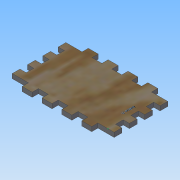
# Autodesk Inventor part: WallToWall(Perpendicular1)
Saved by Autodesk Inventor 2015 (Build 190159000, 159)
## iProperties
Created: 2014-11-11
Part Number: WallToWall(Perpendicular1)
Material: Generic
Document SubType Name: Modeling
Designer: 0
Density: 1 g/cm^3
Appearance: Default
Mass: 72.7404 g
Surface Area: 272.974 cm^2
Volume: 72.7404 cm^3
Author: 0
Autodesk Inventor part; units mm, degrees
ref_plane "YZ Plane" through (0, 0, 0) normal (1, 0, 0) x (0, 1, 0)
ref_plane "XZ Plane" through (0, 0, 0) normal (0, 1, 0) x (-1, 0, 0)
ref_plane "XY Plane" through (0, 0, 0) normal (0, 0, 1) x (1, 0, 0)
sketch "Sketch1" plane through (0, 0, 0) normal (0, 1, 0) x (-1, 0, 0)
  line L0 (0, 0) -> (127, 0)
  line L1 (127, 0) -> (127, -76.2)
  line L2 (127, -76.2) -> (0, -76.2)
  line L3 (0, -76.2) -> (0, 0)
  dimension "BoxHeight" = 127
  dimension "d1" = 76.2
  constraints: 8 end point, 2 parallel, 1 coincident, 1 horizontal, 1 perpendicular
  measures "BoxHeight" distance of L1.end L2.end
  measures "d1" distance of L0.end L1.end
sketch "Sketch2" plane through (0, 0, 0) normal (0, 1, 0) x (-1, 0, 0)
  line L0 (0, 0) -> (-8.89, 0)
  line L1 (-8.89, 0) -> (-8.89, -10.8857)
  line L2 (-8.89, -10.8857) -> (0, -10.8857)
  line L3 (0, -10.8857) -> (0, 0)
  line L4 (0, -76.2) -> (0, 0) projected
  line L5 (0, 0) -> (127, 0) projected
  line L6 (0, -21.7714) -> (-8.89, -21.7714)
  line L7 (-8.89, -21.7714) -> (-8.89, -32.6571)
  line L8 (-8.89, -32.6571) -> (0, -32.6571)
  line L9 (0, -32.6571) -> (0, -21.7714)
  line L10 (0, -43.5429) -> (-8.89, -43.5429)
  line L11 (-8.89, -43.5429) -> (-8.89, -54.4286)
  line L12 (-8.89, -54.4286) -> (0, -54.4286)
  line L13 (0, -54.4286) -> (0, -43.5429)
  line L14 (63.5, 0) -> (63.5, -115.824) construction
  line L15 (127, -10.8857) -> (127, 0)
  line L16 (127, -76.2) -> (127, 0)
  line L17 (127, -32.6571) -> (127, -21.7714)
  line L18 (127, -54.4286) -> (127, -43.5429)
  line L19 (28.2222, -76.2) -> (14.1111, -76.2)
  line L20 (14.1111, -76.2) -> (14.1111, -85.09)
  line L21 (14.1111, -85.09) -> (28.2222, -85.09)
  line L22 (28.2222, -85.09) -> (28.2222, -76.2)
  line L23 (127, -76.2) -> (0, -76.2) projected
  line L24 (56.4444, -76.2) -> (42.3333, -76.2)
  line L25 (42.3333, -76.2) -> (42.3333, -85.09)
  line L26 (42.3333, -85.09) -> (56.4444, -85.09)
  line L27 (56.4444, -85.09) -> (56.4444, -76.2)
  line L28 (84.6667, -76.2) -> (70.5556, -76.2)
  line L29 (70.5556, -76.2) -> (70.5556, -85.09)
  line L30 (70.5556, -85.09) -> (84.6667, -85.09)
  line L31 (84.6667, -85.09) -> (84.6667, -76.2)
  line L32 (112.8889, -76.2) -> (98.7778, -76.2)
  line L33 (98.7778, -76.2) -> (98.7778, -85.09)
  line L34 (98.7778, -85.09) -> (112.8889, -85.09)
  line L35 (112.8889, -85.09) -> (112.8889, -76.2)
  line L36 (127, -38.1) -> (0, -38.1) construction
  line L37 (63.5, -76.2) -> (63.5, 39.624) construction
  line L38 (28.2222, 0) -> (14.1111, 0)
  line L39 (14.1111, 0) -> (14.1111, 8.89)
  line L40 (14.1111, 8.89) -> (28.2222, 8.89)
  line L41 (28.2222, 8.89) -> (28.2222, 0)
  line L42 (127, 0) -> (0, 0)
  line L43 (56.4444, 0) -> (42.3333, 0)
  line L44 (42.3333, 0) -> (42.3333, 8.89)
  line L45 (42.3333, 8.89) -> (56.4444, 8.89)
  line L46 (56.4444, 8.89) -> (56.4444, 0)
  line L47 (84.6667, 0) -> (70.5556, 0)
  line L48 (70.5556, 0) -> (70.5556, 8.89)
  line L49 (84.6667, 8.89) -> (84.6667, 0)
  line L50 (70.5556, 8.89) -> (84.6667, 8.89)
  line L51 (112.8889, 0) -> (98.7778, 0)
  line L52 (98.7778, 0) -> (98.7778, 8.89)
  line L53 (112.8889, 8.89) -> (112.8889, 0)
  line L54 (98.7778, 8.89) -> (112.8889, 8.89)
  line L55 (0, -65.3143) -> (-8.89, -65.3143)
  line L56 (-8.89, -65.3143) -> (-8.89, -76.2)
  line L57 (-8.89, -76.2) -> (0, -76.2)
  line L58 (0, -76.2) -> (0, -65.3143)
  line L59 (127, 0) -> (135.89, 0)
  line L60 (135.89, 0) -> (135.89, -10.8857)
  line L61 (135.89, -10.8857) -> (127, -10.8857)
  line L62 (127, -10.8857) -> (127, 0)
  line L63 (127, -76.2) -> (127, 0)
  line L64 (127, -21.7714) -> (135.89, -21.7714)
  line L65 (135.89, -21.7714) -> (135.89, -32.6571)
  line L66 (135.89, -32.6571) -> (127, -32.6571)
  line L67 (127, -32.6571) -> (127, -21.7714)
  line L68 (127, -43.5429) -> (135.89, -43.5429)
  line L69 (135.89, -43.5429) -> (135.89, -54.4286)
  line L70 (135.89, -54.4286) -> (127, -54.4286)
  line L71 (127, -54.4286) -> (127, -43.5429)
  line L72 (135.89, -65.3143) -> (135.89, -76.2)
  line L73 (127, -65.3143) -> (135.89, -65.3143)
  line L74 (135.89, -76.2) -> (127, -76.2)
  line L75 (127, -76.2) -> (127, -65.3143)
  dimension "d2" = 8.89
  dimension "d3" = 10.8857
  dimension "d5" = 8.89
  dimension "d6" = 10.8857
  dimension "d7" = 10.8857
  dimension "d8" = 8.89
  dimension "d9" = 10.8857
  dimension "d10" = 10.8857
  dimension "d11" = 14.1111
  dimension "d12" = 127
  dimension "d13" = 14.1111
  dimension "d14" = 8.89
  dimension "d15" = 8.89
  dimension "d16" = 14.1111
  dimension "d17" = 8.89
  dimension "d18" = 14.1111
  dimension "d22" = 8.89
  dimension "d23" = 14.1111
  dimension "d27" = 14.1111
  dimension "d28" = 14.1111
  dimension "d29" = 14.1111
  dimension "d34" = 76.2
  dimension "d35" = 8.89
  dimension "d36" = 10.8857
  dimension "d41" = 10.8857
  constraints: 146 end point, 41 symmetric about line, 16 parallel, 9 collinear, 8 horizontal, 8 perpendicular, 2 midpoint, 1 vertical
  measures "d2" distance of L1.end L2.end
  measures "d3" distance of L0.end L1.end
  measures "d5" distance of L7.end L8.end
  measures "d6" distance of L6.end L7.end
  measures "d7" distance between parallel lines of L2 L6
  measures "d8" distance of L10.start L10.end
  measures "d9" distance of L10.end L11.end
  measures "d10" distance between parallel lines of L8 L10
  measures "d11" distance between parallel lines of L4 L20
  measures "d12" distance of L23.start L4.start
  measures "d13" distance of L20.end L21.end
  measures "d14" distance of L19.end L20.end
  measures "d15" distance of L24.end L25.end
  measures "d16" distance of L25.end L26.end
  measures "d17" distance of L28.end L29.end
  measures "d18" distance of L29.end L31.start
  measures "d22" distance of L32.end L33.end
  measures "d23" distance of L33.end L35.start
  measures "d27" distance between parallel lines of L25 L22
  measures "d28" distance between parallel lines of L27 L29
  measures "d29" distance between parallel lines of L31 L33
  measures "d34" distance of L4.start L4.end
  measures "d35" distance of L55.start L56.start
  measures "d36" distance of L56.start L56.end
  measures "d41" distance between parallel lines of L55 L12
extrude "Connections" add sketch "Sketch2" along normal blind 6.35 contours L3 L2 L1 L0 | L39 L40 L41 L5 | L4 L8 L7 L6 | L44 L45 L46 L5 | L4 L12 L11 L10 | L48 L50 L49 L5 | L4 L57 L56 L55 | L52 L54 L53 L5 | L19 L22 L21 L20 | L59 L60 L61 L15 | L23 L27 L26 L25 | L64 L65 L66 L16 | L23 L31 L30 L29 | L68 L69 L70 L16 | L23 L35 L34 L33 | L73 L72 L74 L16
extrude "Base Extrusion" add sketch "Sketch1" along normal blind 6.35
sketch "Sketch3" plane through (0, 6.35, 0) normal (0, 1, 0) x (1, 0, 0)
  line L0 (-6.6713, 46.5048) -> (-6.6713, 27.1528) construction
  line L1 (-6.6713, 27.1528) -> (-46.955, 27.1528) construction
  line L2 (-46.955, 27.1528) -> (-46.955, 46.5048) construction
  line L3 (-46.955, 46.5048) -> (-6.6713, 46.5048) construction
  point P0 (0, 0)
  constraints: 2 other
sketch "Sketch4" plane through (0, 0, 0) normal (0, -1, 0) x (1, 0, 0)
  line L0 (-84.6667, 8.89) -> (-70.5556, 8.89) projected
  line L1 (-84.6667, 0) -> (-84.6667, 8.89) projected
  line L2 (-84.6667, 0) -> (-98.7778, 0) projected
  line L3 (-98.7778, 0) -> (-98.7778, 8.89) projected
  line L4 (-98.7778, 8.89) -> (-112.8889, 8.89) projected
  line L5 (-112.8889, 8.89) -> (-112.8889, 0) projected
  line L6 (-135.89, 0) -> (-112.8889, 0) projected
  line L7 (-135.89, -10.8857) -> (-135.89, 0) projected
  line L8 (-127, -10.8857) -> (-135.89, -10.8857) projected
  line L9 (-127, -10.8857) -> (-127, -21.7714) projected
  line L10 (-135.89, -21.7714) -> (-127, -21.7714) projected
  line L11 (-135.89, -32.6571) -> (-135.89, -21.7714) projected
  line L12 (-127, -32.6571) -> (-135.89, -32.6571) projected
  line L13 (-127, -32.6571) -> (-127, -43.5429) projected
  line L14 (-135.89, -43.5429) -> (-127, -43.5429) projected
  line L15 (-135.89, -54.4286) -> (-135.89, -43.5429) projected
  line L16 (-127, -54.4286) -> (-135.89, -54.4286) projected
  line L17 (-127, -54.4286) -> (-127, -65.3143) projected
  line L18 (-127, -65.3143) -> (-135.89, -65.3143) projected
  line L19 (-135.89, -65.3143) -> (-135.89, -76.2) projected
  line L20 (-135.89, -76.2) -> (-112.8889, -76.2) projected
  line L21 (-112.8889, -76.2) -> (-112.8889, -85.09) projected
  line L22 (-112.8889, -85.09) -> (-98.7778, -85.09) projected
  line L23 (-98.7778, -85.09) -> (-98.7778, -76.2) projected
  line L24 (-98.7778, -76.2) -> (-84.6667, -76.2) projected
  line L25 (-84.6667, -76.2) -> (-84.6667, -85.09) projected
  line L26 (-84.6667, -85.09) -> (-70.5556, -85.09) projected
  line L27 (-70.5556, -85.09) -> (-70.5556, -76.2) projected
  line L28 (-70.5556, -76.2) -> (-56.4444, -76.2) projected
  line L29 (-56.4444, -85.09) -> (-56.4444, -76.2) projected
  line L30 (-42.3333, -85.09) -> (-56.4444, -85.09) projected
  line L31 (-42.3333, -76.2) -> (-42.3333, -85.09) projected
  line L32 (-42.3333, -76.2) -> (-28.2222, -76.2) projected
  line L33 (-28.2222, -85.09) -> (-28.2222, -76.2) projected
  line L34 (-14.1111, -85.09) -> (-28.2222, -85.09) projected
  line L35 (-14.1111, -76.2) -> (-14.1111, -85.09) projected
  line L36 (-14.1111, -76.2) -> (8.89, -76.2) projected
  line L37 (8.89, -76.2) -> (8.89, -65.3143) projected
  line L38 (8.89, -65.3143) -> (0, -65.3143) projected
  line L39 (0, -65.3143) -> (0, -54.4286) projected
  line L40 (8.89, -54.4286) -> (0, -54.4286) projected
  line L41 (8.89, -43.5429) -> (8.89, -54.4286) projected
  line L42 (0, -43.5429) -> (8.89, -43.5429) projected
  line L43 (0, -43.5429) -> (0, -32.6571) projected
  line L44 (8.89, -32.6571) -> (0, -32.6571) projected
  line L45 (8.89, -21.7714) -> (8.89, -32.6571) projected
  line L46 (0, -21.7714) -> (8.89, -21.7714) projected
  line L47 (0, -21.7714) -> (0, -10.8857) projected
  line L48 (8.89, -10.8857) -> (0, -10.8857) projected
  line L49 (8.89, 0) -> (8.89, -10.8857) projected
  line L50 (-14.1111, 0) -> (8.89, 0) projected
  line L51 (-14.1111, 0) -> (-14.1111, 8.89) projected
  line L52 (-14.1111, 8.89) -> (-28.2222, 8.89) projected
  line L53 (-28.2222, 8.89) -> (-28.2222, 0) projected
  line L54 (-28.2222, 0) -> (-42.3333, 0) projected
  line L55 (-42.3333, 8.89) -> (-42.3333, 0) projected
  line L56 (-56.4444, 8.89) -> (-42.3333, 8.89) projected
  line L57 (-56.4444, 0) -> (-56.4444, 8.89) projected
  line L58 (-56.4444, 0) -> (-70.5556, 0) projected
  line L59 (-70.5556, 8.89) -> (-70.5556, 0) projected
  point P0 (0, 0)
equation "\"d1\" = BaseLength"
equation "\"d2\" = PerpA"
equation "\"d3\" = PerpB"
equation "\"d5\" = d2"
equation "\"d6\" = d3"
equation "\"d7\" = PerpSpace"
equation "\"d8\" = d2"
equation "\"d9\" = d3"
equation "\"d10\" = d7"
equation "\"d11\" = -0.8 * d13 + 0.2 * d12"
equation "\"d13\" = 0.111111 * d12"
equation "\"d14\" = WallConA"
equation "\"d15\" = d14"
equation "\"d16\" = d13"
equation "\"d17\" = d15"
equation "\"d18\" = d20"
equation "\"d22\" = d14"
equation "\"d23\" = d25"
equation "\"d27\" = d11"
equation "\"d28\" = d27"
equation "\"d29\" = d11"
equation "\"d35\" = d37"
equation "\"d36\" = d38"
equation "\"d41\" = d10"
equation "\"d20\" = 0.111111 * d21"
equation "\"d25\" = 0.111111 * d26"
equation "\"d37\" = d39"
equation "\"d38\" = d40"
equation "\"BaseLength\" = 76.2"
equation "\"PerpA\" = 8.89"
equation "\"PerpB\" = 10.885714"
equation "\"PerpSpace\" = 10.885714"
equation "\"WallConA\" = 8.89"
equation "\"d21\" = 127"
equation "\"d26\" = 127"
equation "\"d39\" = 8.89"
equation "\"d40\" = 10.885714"
body "Solid1"
